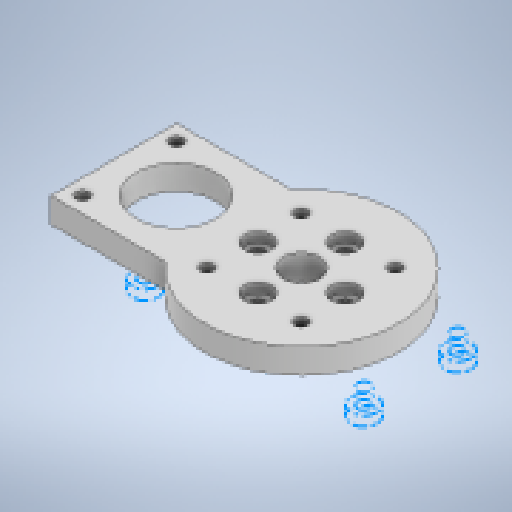
# Autodesk Inventor part: gripper_6&7_connector
Saved by Autodesk Inventor 2024 (Build 280153000, 153)
## iProperties
Created: 2023-09-23
Part Number: gripper_6&7_connector
Material: Generic
Document SubType Name: Modeling
Designer: 박동준
Density: 1 g/cm^3
Appearance: Default
Author: 박동준
Autodesk Inventor part; units mm, degrees
ref_plane "YZ Plane" through (0, 0, 0) normal (1, 0, 0) x (0, 1, 0)
ref_plane "XZ Plane" through (0, 0, 0) normal (0, 1, 0) x (-1, 0, 0)
ref_plane "XY Plane" through (0, 0, 0) normal (0, 0, 1) x (1, 0, 0)
sketch "Sketch1" plane through (0, 0, 0) normal (0, 1, 0) x (-1, 0, 0)
  line L0 (20.05, -10.07) -> (-20.05, -10.07)
  line L1 (-20.05, -10.07) -> (-20.05, 10.07)
  line L2 (-20.05, 10.07) -> (20.05, 10.07)
  line L3 (20.05, 10.07) -> (20.05, -10.07)
  point P0 (0, 0)
  point P1 (0, -10.07)
  point P2 (20.05, 0)
  dimension "d0" = 40.1
  dimension "d1" = 20.14
  constraints: 8 end point, 2 midpoint, 2 parallel, 1 horizontal, 1 horizontal alignment, 1 perpendicular, 1 vertical alignment
  measures "d0" distance of L0.start L0.end
  measures "d1" distance of L2.end L0.start
extrude "Extrusion1" add sketch "Sketch1" along normal blind 4
sketch "Sketch3" plane through (0, 0, 0) normal (0, -1, 0) x (1, 0, 0)
  ellipse E0 centre (-17.932, 7.952) end of major axis (-18.798, 8.818) minor radius 1 (-18.1556, 9.07) -> (-19.05, 8.1756) ccw projected
  line L0 (-19.05, -8.1756) -> (-19.05, 8.1756) projected
  ellipse E1 centre (-17.932, -7.952) end of major axis (-18.798, -8.818) minor radius 1 (-19.05, -8.1756) -> (-18.1556, -9.07) ccw projected
  line L1 (18.1556, -9.07) -> (-18.1556, -9.07) projected
  ellipse E2 centre (17.932, -7.952) end of major axis (18.798, -8.818) minor radius 1 (18.1556, -9.07) -> (19.05, -8.1756) ccw projected
  line L2 (19.05, 8.1756) -> (19.05, -8.1756) projected
  ellipse E3 centre (17.932, 7.952) end of major axis (18.798, 8.818) minor radius 1 (19.05, 8.1756) -> (18.1556, 9.07) ccw projected
  line L3 (-18.1556, 9.07) -> (18.1556, 9.07) projected
  circle A0 centre (17.55, -7.525) radius 0.7835 projected
  circle A1 centre (17.55, 7.525) radius 0.7835 projected
  circle A2 centre (2.45, -7.525) radius 0.7835 projected
  circle A3 centre (2.45, 7.525) radius 0.7835 projected
  circle A4 centre (-17.55, -7.525) radius 0.7835 projected
  circle A5 centre (-17.55, 7.525) radius 0.7835 projected
  circle A6 centre (-10.05, 0) radius 6.4 projected
  circle A7 centre (-10.05, 0) radius 6.5
  point P0 (0, 0)
  dimension "d11" = 13
  constraints: 1 centre point, 1 coincident, 4 other
  measures "d11" diameter of A7
extrude "Extrusion2" cut sketch "Sketch3" against normal through all contours A6
sketch "Sketch7" plane through (0, 0, 0) normal (0, -1, 0) x (1, 0, 0)
  line L0 (16.15, -10.17) -> (-0.9759, -10.17) projected
  arc A0 (-0.9759, -10.17) -> (-0.9759, 10.17) centre (10.05, 0) ccw projected
  line L1 (-0.9759, 10.17) -> (16.15, 10.17) projected
  line L2 (16.15, 10.17) -> (16.15, 8.07) projected
  arc A1 (16.15, 8.07) -> (18.05, 6.17) centre (18.05, 8.07) ccw projected
  line L3 (18.05, 6.17) -> (20.15, 6.17) projected
  line L4 (20.15, 6.17) -> (20.15, -6.17) projected
  line L5 (20.15, -6.17) -> (18.05, -6.17) projected
  arc A2 (18.05, -6.17) -> (16.15, -8.07) centre (18.05, -8.07) ccw projected
  line L6 (16.15, -8.07) -> (16.15, -10.17) projected
  circle A3 centre (10.05, 0) radius 15.5
  circle A4 centre (-10.05, 0) radius 6.4 projected
  circle A5 centre (-10.05, 0) radius 6.4
  point P0 (0, 0)
  point P1 (-4.9575, 3.8763)
  point P2 (-4.9575, -3.8763)
  dimension "d31" = 31
  constraints: 2 centre point, 2 coincident, 1 concentric
  measures "d31" diameter of A3
extrude "Extrusion4" add sketch "Sketch7" against normal up to surface (4 mm away) contours L6 A2 L5 L4 L3 A1 L2 L1 A0 L0 | A3 A4 picked at (9.8263, 0)
sketch "Sketch8" plane through (0, 4, 0) normal (0, 1, 0) x (1, 0, 0)
  circle A0 centre (10.05, 7) radius 0.7835 projected
  circle A1 centre (17.05, 0) radius 0.7835 projected
  circle A2 centre (10.05, -7) radius 0.7835 projected
  circle A3 centre (3.05, 0) radius 0.7835 projected
  circle A4 centre (10.05, 0) radius 1.75 projected
  circle A5 centre (10.05, 0) radius 9.96 projected
  point P0 (0, 0)
hole "Hole4" at (10.05, 4, 7) at (3.05, 4, 0) at (17.05, 4, 0) at (10.05, 4, -7) direction (0, -1, 0) diameter 2.1 end through all counterbore diameter 4.3 counterbore depth 1.5
sketch "Sketch9" plane through (0, 4, 0) normal (0, 1, 0) x (1, 0, 0)
  circle A0 centre (10.05, 0) radius 4.5 projected
  circle A1 centre (10.05, 0) radius 2.925 projected
  circle A2 centre (10.05, 0) radius 2.975
  point P0 (0, 0)
  dimension "d41" = 5.95
  constraints: 1 centre point, 1 coincident
  measures "d41" diameter of A2
extrude "Extrusion5" cut sketch "Sketch9" against normal through all contours A1 | A2
sketch "Sketch10" plane through (0, 0, 0) normal (0, -1, 0) x (1, 0, 0)
  ellipse E0 centre (-17.932, 7.952) end of major axis (-18.798, 8.818) minor radius 1 (-18.1556, 9.07) -> (-19.05, 8.1756) ccw projected
  line L0 (-19.05, -8.1756) -> (-19.05, 8.1756) projected
  ellipse E1 centre (-17.932, -7.952) end of major axis (-18.798, -8.818) minor radius 1 (-19.05, -8.1756) -> (-18.1556, -9.07) ccw projected
  line L1 (18.1556, -9.07) -> (-18.1556, -9.07) projected
  ellipse E2 centre (17.932, -7.952) end of major axis (18.798, -8.818) minor radius 1 (18.1556, -9.07) -> (19.05, -8.1756) ccw projected
  line L2 (19.05, 8.1756) -> (19.05, -8.1756) projected
  ellipse E3 centre (17.932, 7.952) end of major axis (18.798, 8.818) minor radius 1 (19.05, 8.1756) -> (18.1556, 9.07) ccw projected
  line L3 (-18.1556, 9.07) -> (18.1556, 9.07) projected
  circle A0 centre (17.55, -7.525) radius 0.7835 projected
  circle A1 centre (17.55, 7.525) radius 0.7835 projected
  circle A2 centre (2.45, -7.525) radius 0.7835 projected
  circle A3 centre (2.45, 7.525) radius 0.7835 projected
  circle A4 centre (-17.55, -7.525) radius 0.7835 projected
  circle A5 centre (-17.55, 7.525) radius 0.7835 projected
  circle A6 centre (-10.05, 0) radius 6.4 projected
  point P0 (0, 0)
  constraints: 4 other
hole "Hole5" at (17.55, 0, -7.525) at (2.45, 0, -7.525) at (-17.55, 0, -7.525) at (17.55, 0, 7.525) at (2.45, 0, 7.525) at (-17.55, 0, 7.525) direction (0, 1, 0) diameter 2.1 end through all counterbore diameter 4.3 counterbore depth 1.5
body "Solid1"
